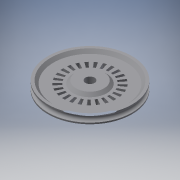
# Autodesk Inventor part: wheel
Saved by Autodesk Inventor 2016 (Build 200138000, 138)
## iProperties
Created: 2016-09-24
Part Number: wheel
Material: Generic
Document SubType Name: Modeling
Designer: benja
Density: 1 g/cm^3
Appearance: Default
Author: benja
Autodesk Inventor part; units mm, degrees
ref_plane "YZ Plane" through (0, 0, 0) normal (1, 0, 0) x (0, 1, 0)
ref_plane "XZ Plane" through (0, 0, 0) normal (0, 1, 0) x (-1, 0, 0)
ref_plane "XY Plane" through (0, 0, 0) normal (0, 0, 1) x (1, 0, 0)
sketch "Sketch1" plane through (0, 0, 0) normal (0, 0, 1) x (1, 0, 0)
  circle A0 centre (0, 0) radius 0.5 projected
  circle A1 centre (0, 0) radius 5
  arc A2 (2.3707, -0.6182) -> (3.6286, -0.9463) centre (2.9997, -0.7822) ccw
  arc A3 (2.3707, -0.6182) -> (2.2208, 1.0347) centre (0, 0) ccw
  arc A4 (3.3992, 1.5837) -> (2.2208, 1.0347) centre (2.81, 1.3092) ccw
  arc A5 (3.6286, -0.9463) -> (3.3992, 1.5837) centre (0, 0) ccw
  arc A6 (2.1772, -0.5678) -> (2.0395, 0.9502) centre (0, 0) ccw
  arc A7 (2.1772, -0.5678) -> (3.8222, -0.9967) centre (2.9997, -0.7822) ccw
  arc A8 (3.8222, -0.9967) -> (3.5805, 1.6681) centre (0, 0) ccw
  arc A9 (3.5805, 1.6681) -> (2.0395, 0.9502) centre (2.81, 1.3092) ccw
  point P0 (0, 0)
  dimension "d1" = 10
  dimension "d48" = 0.2
  constraints: 16 point on circle, 9 centre point, 1 concentric, 15 other
  measures "d1" diameter of A1
  measures "d48" radial gap between concentric circles of A3 A6
extrude "Extrusion1" add sketch "Sketch1" along normal blind 2.3 contours A0 | A1
sketch "Sketch2" plane through (0, 0, 2.3) normal (0, 0, 1) x (1, 0, 0)
  circle A0 centre (0, 0) radius 5 projected
  point P0 (0, 0)
extrude "Extrusion2" add sketch "Sketch2" along normal blind 3.7
sketch "Sketch3" plane through (0, 0, 0) normal (0, 1, 0) x (-1, 0, 0)
  line L0 (5, 6) -> (-5, 6) projected
  line L1 (-5, 0) -> (5, 0) projected
  line L2 (5, 6) -> (-5, 6) projected
  line L3 (-15, 3) -> (-5, 3)
  line L4 (-5, 0) -> (-5, 6) projected
  line L5 (-5, 6) -> (-5, 5.9384)
  line L6 (-5, 0) -> (5, 0) projected
  line L7 (0, -1.6) -> (0, 9.6) projected
  arc A0 (-15, 3.5) -> (-15, 5.5) centre (-15, 4.5) ccw
  line L8 (-15, 6) -> (-15, 5.5)
  line L9 (-15, 3.5) -> (-15, 3)
  line L10 (-15, 6) -> (-14, 6)
  line L11 (-14, 6) -> (-13, 5)
  line L12 (-13, 5) -> (-5, 5)
  point P0 (0, 0)
  point P1 (-13, 3)
  point P2 (-5, 3.5)
  dimension "d9" = 3
  dimension "d10" = 3
  dimension "d23" = 2
  dimension "d25" = 15
  dimension "d38" = 2
  dimension "d39" = 1
  dimension "d40" = 135
  constraints: 14 end point, 4 perpendicular, 4 point on line, 3 collinear, 2 parallel, 2 point on circle, 1 centre point, 1 midpoint
  measures "d9" distance of L8.start L3.start
  measures "d10" distance between parallel lines of L6 L3
  measures "d23" diameter of A0
  measures "d25" distance between parallel lines of L7 L9
  measures "d38" distance between parallel lines of L3 L12
  measures "d39" horizontal distance of A0.centre L10.end
  measures "d40" angle of L10 L11
revolve "Revolution1" add sketch "Sketch3" angle 360 about axis through (0, 0, -10) along (0, 0, 1) contours L4 L3 L9 A0 L8 L10 L11 L12
hole "Hole1" at (0, 0, 6) direction (0, 0, -1) diameter 3.3 depth 5
chamfer "Chamfer2" distance 1 angle 45 1 edges at (-5, 0, 5)
sketch "Sketch5" plane through (0, 0, 5) normal (0, 0, 1) x (1, 0, 0)
  arc A0 (-0.3908, -6.9891) -> (0.3908, -6.9891) centre (0, 0) ccw
  arc A1 (-0.5303, -9.4852) -> (0.5303, -9.4852) centre (0, 0) ccw
  line L0 (0.3908, -6.9891) -> (0.5303, -9.4852)
  line L1 (-0.3908, -6.9891) -> (-0.5303, -9.4852)
  line L2 (0, 0) -> (0, -10.4532) construction
  circle A2 centre (0, 0) radius 6 projected
  dimension "d58" = 3.2
  dimension "d59" = 6.4
  dimension "d60" = 2.5
  dimension "d61" = 7
  constraints: 6 end point, 4 point on circle, 2 centre point, 2 coincident, 2 point on line, 1 vertical
  measures "d58" angle of L0 L2
  measures "d59" angle of L1 L0
  measures "d60" radial gap between concentric circles of A1 A0
  measures "d61" radius of A0
extrude "Extrusion4" cut sketch "Sketch5" against normal up to next contours A0 L0 A1 L1
pattern_circular "Circular Pattern2" count 25 over 360 about axis through (0, 0, 3.5) along (0, 0, 1) of "Extrusion4"
equation "\"d58\" = 0.5 * d59"
body "Solid1"
